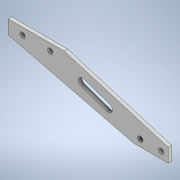
# Autodesk Inventor part: arm_2
Saved by Autodesk Inventor 2020 (Build 240168000, 168)
## iProperties
Created: 2020-01-20
Part Number: arm_2
Material: Generic
Document SubType Name: Modeling
Designer: psrobotics
Density: 1 g/cm^3
Appearance: Default
Author: psrobotics
Autodesk Inventor part; units mm, degrees
ref_plane "YZ Plane" through (0, 0, 0) normal (1, 0, 0) x (0, 1, 0)
ref_plane "XZ Plane" through (0, 0, 0) normal (0, 1, 0) x (-1, 0, 0)
ref_plane "XY Plane" through (0, 0, 0) normal (0, 0, 1) x (1, 0, 0)
sketch "Sketch1" plane through (0, 0, 0) normal (0, 0, 1) x (1, 0, 0)
  line L0 (-158.3346, -22.9633) -> (-158.3346, -15.0367) projected
  arc A0 (-32.2589, 3) -> (-35, 2.3373) centre (-32.2589, -3) ccw projected
  line L1 (-35, 2.3373) -> (-35, -5) projected
  line L2 (0, -5) -> (-35, -5) projected
  line L3 (0, 3) -> (0, -5) projected
  line L4 (0, 3) -> (-32.2589, 3) projected
  circle A1 centre (-8, -1) radius 2 projected
  circle A2 centre (-24, -1) radius 2 projected
  line L5 (-158.3346, -19) -> (0, -19)
  line L6 (-64, 3) -> (-56, 3) projected
  line L7 (-60, 3) -> (-60, 13)
  line L8 (-60, 13) -> (70, 13)
  line L9 (-32.2589, 3) -> (-32.2589, -5)
  line L10 (70, 13) -> (70, -19)
  line L11 (70, -19) -> (60, -19)
  line L12 (60, -19) -> (50, -19)
  line L13 (40, -15) -> (60, -15)
  line L14 (60, -15) -> (60, -23)
  line L15 (60, -23) -> (40, -23)
  line L16 (40, -23) -> (40, -15)
  line L17 (40, -15) -> (60, -23) construction
  line L18 (60, -15) -> (40, -23) construction
  line L19 (0, 3) -> (60, -15)
  line L20 (50, -19) -> (44, -19)
  circle A3 centre (44, -19) radius 1.5
  line L21 (50, -19) -> (56, -19)
  circle A4 centre (56, -19) radius 1.5
  line L22 (-32.2589, -5) -> (40, -23)
  point P0 (0, 0)
  dimension "d0" = 10
  dimension "d1" = 130
  dimension "d2" = 32
  dimension "d3" = 10
  dimension "d4" = 10
  dimension "d5" = 20
  dimension "d6" = 8
  dimension "d7" = 6
  dimension "d8" = 3
  dimension "d9" = 6
  dimension "d10" = 3
  constraints: 34 end point, 4 horizontal, 4 midpoint, 4 parallel, 3 perpendicular, 2 centre point, 2 coincident, 2 point on line, 1 vertical
  measures "d0" distance of L7.start L7.end
  measures "d1" distance of L7.end L8.end
  measures "d2" distance of L8.end L10.end
  measures "d3" distance of L10.end L11.end
  measures "d4" distance of L11.end L12.end
  measures "d5" distance of L13.start L13.end
  measures "d6" distance of L13.end L14.end
  measures "d7" distance of L12.end L20.end
  measures "d8" diameter of A3
  measures "d9" distance of L12.end L21.end
  measures "d10" diameter of A4
extrude "Extrusion1" add sketch "Sketch1" along normal blind 2 contours L4 L3 L2 L9 | L19 L13 L16 L22 L2 L3 | L14 L15 L16 L13
sketch "Sketch3" plane through (0, 0, 0) normal (0, 0, -1) x (-1, 0, 0)
  line L0 (0, 3) -> (32.2589, 3) projected
  line L1 (-60, -15) -> (0, 3) projected
  line L2 (-60, -23) -> (-60, -15) projected
  line L3 (-40, -23) -> (-60, -23) projected
  line L4 (32.2589, -5) -> (-40, -23) projected
  line L5 (32.2589, 3) -> (32.2589, -5) projected
  circle A0 centre (-56, -19) radius 1.5 projected
  circle A1 centre (-44, -19) radius 1.5 projected
  circle A2 centre (24, -1) radius 2 projected
  circle A3 centre (8, -1) radius 2 projected
  circle A4 centre (8, -1) radius 1.5
  circle A5 centre (24, -1) radius 1.5
  point P0 (0, 0)
  dimension "d23" = 3
  dimension "d24" = 3
  constraints: 2 centre point, 2 coincident
  measures "d23" diameter of A4
  measures "d24" diameter of A5
extrude "Extrusion3" add sketch "Sketch3" against normal blind 2 contours A2 | A3
sketch "Sketch4" plane through (0, 0, 2) normal (0, 0, 1) x (1, 0, 0)
  circle A0 centre (-24, -1) radius 1.5 projected
  circle A1 centre (-8, -1) radius 1.5 projected
  line L0 (-32.2589, 3) -> (-32.2589, -5) projected
  line L1 (-32.2589, -5) -> (40, -23) projected
  line L2 (40, -23) -> (60, -23) projected
  line L3 (60, -23) -> (60, -15) projected
  line L4 (60, -15) -> (0, 3) projected
  line L5 (0, 3) -> (-32.2589, 3) projected
  circle A2 centre (56, -19) radius 1.5 projected
  circle A3 centre (44, -19) radius 1.5 projected
  circle A4 centre (-8, -1) radius 1.5 projected
  line L6 (-8, -1) -> (44, -19)
  line L7 (10.4401, -7.3831) -> (25.5599, -12.6169) construction
  line L8 (9.7041, -9.5093) -> (24.8239, -14.7431)
  line L9 (26.2959, -10.4907) -> (11.1761, -5.2569)
  arc A5 (11.1761, -5.2569) -> (9.7041, -9.5093) centre (10.4401, -7.3831) ccw
  arc A6 (24.8239, -14.7431) -> (26.2959, -10.4907) centre (25.5599, -12.6169) ccw
  point P0 (0, 0)
  point P1 (18, -10)
  dimension "d27" = 8
  dimension "d28" = 4.5
  constraints: 10 end point, 4 point on circle, 4 tangent, 2 centre point, 2 midpoint, 1 parallel, 1 point on line
  measures "d27" distance of point (18, -10) L7.end
  measures "d28" diameter of A6
extrude "Extrusion4" cut sketch "Sketch4" against normal blind 10 contours A5 L9 A6 L6 | L6 A6 L8 A5
body "Solid1"
